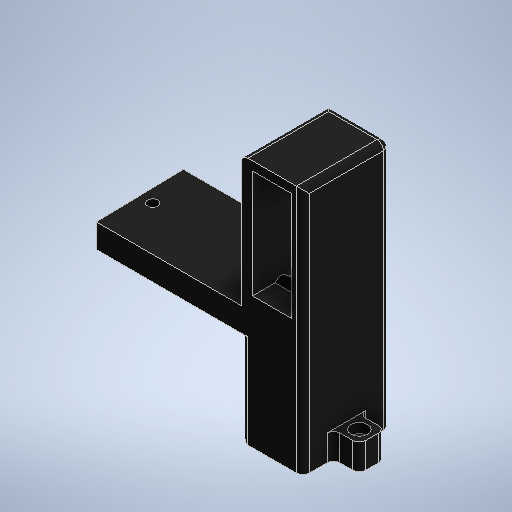
# Autodesk Inventor part: Servo Housing
Saved by Autodesk Inventor 2025.4 (Build 294407000, 407)
## iProperties
Created: 2026-05-20
Part Number: Servo Housing
Material: Generic
Document SubType Name: Modeling
Designer: lenovo
Density: 1 g/cm^3
Appearance: Default(1)
Author: lenovo
Autodesk Inventor part; units mm, degrees
ref_plane "YZ Plane" through (0, 0, 0) normal (1, 0, 0) x (0, 1, 0)
ref_plane "XZ Plane" through (0, 0, 0) normal (0, 1, 0) x (-1, 0, 0)
ref_plane "XY Plane" through (0, 0, 0) normal (0, 0, 1) x (1, 0, 0)
sketch "Sketch1" plane through (0, 0, 0) normal (0, 0, 1) x (1, 0, 0)
  line L0 (-9.5, 19.5) -> (9.5, 19.5)
  line L1 (9.5, 19.5) -> (9.5, -19.5)
  line L2 (9.5, -19.5) -> (-9.5, -19.5)
  line L3 (-9.5, -19.5) -> (-9.5, 19.5)
  line L4 (-9.5, 19.5) -> (9.5, -19.5) construction
  line L5 (9.5, 19.5) -> (-9.5, -19.5) construction
  point P0 (0, 0)
  dimension "d0" = 19
  dimension "d1" = 39
  constraints: 12 end point, 2 midpoint, 2 parallel, 1 horizontal, 1 perpendicular
  measures "d0" distance of L1.end L2.end
  measures "d1" distance of L0.end L1.end
extrude "Extrusion1" add sketch "Sketch1" along normal mid plane 27
sketch "Sketch2" plane through (0, 0, 13.5) normal (0, 0, 1) x (1, 0, 0)
  line L0 (-6.075, 16.75) -> (6.075, 16.75)
  line L1 (6.075, 16.75) -> (6.075, -16.75)
  line L2 (6.075, -16.75) -> (-6.075, -16.75)
  line L3 (-6.075, -16.75) -> (-6.075, 16.75)
  line L4 (-6.075, 16.75) -> (6.075, -16.75) construction
  line L5 (6.075, 16.75) -> (-6.075, -16.75) construction
  point P0 (0, 0)
  dimension "d4" = 12.15
  dimension "d5" = 33.5
  constraints: 12 end point, 2 midpoint, 2 parallel, 1 horizontal, 1 perpendicular
  measures "d4" distance of L1.end L2.end
  measures "d5" distance of L0.end L1.end
extrude "Extrusion2" cut sketch "Sketch2" against normal blind 7
sketch "Sketch3" plane through (0, 0, 6.5) normal (0, 0, 1) x (1, 0, 0)
  line L0 (-6.075, -16.75) -> (-6.075, 16.75) projected
  line L1 (-6.075, 0) -> (6.075, 0)
  line L2 (6.075, 16.75) -> (6.075, -16.75) projected
  circle A0 centre (0, 13.875) radius 0.625
  circle A1 centre (0, -13.875) radius 0.625
  line L3 (6.075, -16.75) -> (-6.075, -16.75) projected
  line L4 (-6.075, -16.75) -> (-4, -12.75)
  line L5 (-4, -12.75) -> (0, -12.75)
  line L6 (-6.075, 16.75) -> (6.075, 16.75) projected
  line L7 (0, 16.75) -> (0, -16.75)
  line L8 (6.075, -16.75) -> (4, -12.75)
  line L9 (4, -12.75) -> (0, -12.75)
  line L10 (-6.075, 16.75) -> (-4, 12.75)
  line L11 (-4, 12.75) -> (0, 12.75)
  line L12 (4, 12.75) -> (0, 12.75)
  line L13 (6.075, 16.75) -> (4, 12.75)
  point P0 (0, 0)
  point P1 (0, 0)
  dimension "d8" = 1.25
  dimension "d9" = 27.75
  dimension "d10" = 4
  dimension "d11" = 4
  constraints: 20 end point, 5 midpoint, 5 symmetric about line, 2 centre point, 2 vertical alignment, 1 parallel, 1 other
  measures "d8" diameter of A0
  measures "d9" diameter of A0.centre L1
  measures "d10" distance of L4.end L5.end
  measures "d11" vertical distance of L0.start L4.end
extrude "Extrusion3" cut sketch "Sketch3" against normal blind 17 contours L0 L1 L7 L5 L4 | L0 L10 L11 L7 L1 | L7 L12 L13 L2 L1 | L1 L2 L8 L9 L7 | L7 A1 | A1 L7 | L7 A0 | A0 L7
sketch "Sketch4" plane through (0, 0, -10.5) normal (0, 0, 1) x (1, 0, 0)
  line L0 (6.075, 16.75) -> (6.075, -16.75) projected
  line L1 (-6.075, -16.75) -> (6.075, -16.75)
  line L2 (6.075, -16.75) -> (6.075, 16.75)
  line L3 (6.075, 16.75) -> (-6.075, 16.75)
  line L4 (-6.075, 16.75) -> (-6.075, -16.75)
  line L5 (-6.075, -16.75) -> (6.075, 16.75) construction
  line L6 (6.075, -16.75) -> (-6.075, 16.75) construction
  point P0 (0, 0)
  constraints: 12 end point, 2 midpoint, 2 parallel, 1 horizontal, 1 perpendicular
extrude "Extrusion4" cut sketch "Sketch4" along normal blind 13
fillet "Fillet1" radius 4 4 edges at (-4, 12.75, 4.5) (4, 12.75, 4.5) (4, -12.75, 4.5) (-4, -12.75, 4.5)
sketch "Sketch5" plane through (0, 0, 13.5) normal (0, 0, 1) x (1, 0, 0)
  line L0 (9.5, -19.5) -> (-9.5, -19.5) projected
  line L1 (-9.5, -19.5) -> (9.5, -19.5)
  line L2 (9.5, -19.5) -> (9.5, -39.5)
  line L3 (9.5, -39.5) -> (-9.5, -39.5)
  line L4 (-9.5, -39.5) -> (-9.5, -19.5)
  point P0 (0, 0)
  point P1 (9.5, -29.5)
  dimension "d18" = 20
  constraints: 8 end point, 2 parallel, 1 horizontal, 1 midpoint, 1 perpendicular, 1 vertical alignment
  measures "d18" distance of L1.end L2.end
extrude "Extrusion5" add sketch "Sketch5" against normal up to surface (27 mm away)
sketch "Sketch6" plane through (-9.5, 19.5, -13.5) normal (-1, 0, 0) x (0, 0, 1)
  line L0 (27, 0) -> (27, -59) projected
  line L1 (0, 0) -> (0, -59) projected
  line L2 (27, -59) -> (27, 0) projected
  line L3 (0, -40) -> (27, -40)
  line L4 (27, -40) -> (27, -48)
  line L5 (27, -48) -> (0, -48)
  line L6 (0, -48) -> (0, -40)
  line L7 (0, 0) -> (27, 0) projected
  point P0 (13.5, -19.5)
  point P1 (27, -29.5)
  point P2 (0, -48)
  dimension "d28" = 8
  dimension "d29" = 40
  constraints: 8 end point, 2 parallel, 2 point on line, 1 horizontal, 1 midpoint, 1 perpendicular
  measures "d28" distance between parallel lines of L3 L5
  measures "d29" distance between parallel lines of L7 L3
extrude "Extrusion6" add sketch "Sketch6" along normal blind 45 contours L0 L5 L1 L3
sketch "Sketch7" plane through (9.5, -39.5, -13.5) normal (0, -1, 0) x (1, 0, 0)
  line L0 (0, 0) -> (0, 27) projected
  line L1 (0, 27) -> (-19, 27)
  line L2 (-19, 27) -> (-19, 0)
  line L3 (-19, 0) -> (0, 0)
  line L4 (0, 0) -> (0, 27)
  point P0 (-9.5, 13.5)
  constraints: 8 end point, 2 parallel, 1 horizontal, 1 perpendicular
extrude "Extrusion7" add sketch "Sketch7" along normal blind 18
sketch "Sketch8" plane through (9.5, -57.5, -13.5) normal (0, -1, 0) x (1, 0, 0)
  line L0 (-15.575, 16) -> (-15.575, 3) projected
  line L1 (-3.425, 16) -> (-15.575, 16) projected
  line L2 (-15.575, 3) -> (-3.425, 3)
  line L3 (-3.425, 3) -> (-3.425, 16)
  line L4 (-3.425, 16) -> (-15.575, 16)
  line L5 (-15.575, 16) -> (-15.575, 3)
  point P0 (-9.5, 13.5)
  constraints: 8 end point, 2 parallel, 1 horizontal, 1 perpendicular
extrude "Extrusion8" cut sketch "Sketch8" against normal up to next
sketch "Sketch9" plane through (9.5, -57.5, -13.5) normal (0, -1, 0) x (1, 0, 0)
  line L0 (0, 0) -> (0, 27) projected
  line L1 (0, 17.5) -> (8, 17.5)
  line L2 (8, 17.5) -> (8, 9.5)
  line L3 (8, 9.5) -> (0, 9.5)
  line L4 (0, 9.5) -> (0, 17.5)
  circle A0 centre (4, 13.5) radius 1.6
  line L5 (-15.575, 16) -> (-3.425, 16) projected
  line L6 (-9.5, 16) -> (-9.5, 3)
  line L7 (-3.425, 3) -> (-15.575, 3) projected
  line L8 (-19, 17.5) -> (-27, 17.5)
  line L9 (-27, 17.5) -> (-27, 9.5)
  line L10 (-27, 9.5) -> (-19, 9.5)
  circle A1 centre (-23, 13.5) radius 1.6
  line L11 (-19, 17.5) -> (-19, 9.5)
  point P0 (-9.5, 13.5)
  point P1 (8, 13.5)
  point P2 (0, 13.5)
  point P3 (4, 17.5)
  point P4 (0, 9.5)
  dimension "d30" = 8
  dimension "d31" = 8
  dimension "d32" = 3.2
  constraints: 18 end point, 5 midpoint, 5 symmetric about line, 2 centre point, 2 horizontal alignment, 2 parallel, 2 perpendicular, 1 horizontal, 1 point on line, 1 vertical alignment, 1 other
  measures "d30" distance of L1.start L1.end
  measures "d31" distance between parallel lines of L1 L3
  measures "d32" diameter of A0
extrude "Extrusion9" add sketch "Sketch9" against normal blind 8
sketch "Sketch10" plane through (9.5, -49.5, -13.5) normal (0, 1, 0) x (1, 0, 0)
  circle A0 centre (4, -13.5) radius 1.6 projected
  circle A1 centre (4, -13.5) radius 2.6
  circle A2 centre (-23, -13.5) radius 2.6
  circle A3 centre (-23, -13.5) radius 1.6 projected
  point P0 (-9.5, -13.5)
  dimension "d35" = 5.2
  dimension "d36" = 5.2
  constraints: 2 centre point, 1 coincident, 1 concentric
  measures "d35" diameter of A1
  measures "d36" diameter of A2
extrude "Extrusion10" cut sketch "Sketch10" against normal blind 3
fillet "Fillet2" radius 2 15 edges at (-9.5, -43, 13.5) (9.5, -19, 13.5) (9.5, -53.5, 4) (17.5, -53.5, 4) (17.5, -53.5, -4) (9.5, -53.5, -4) (6.075, -20.375, -10.5) (-9.5, -43, -13.5) (-9.5, -53.5, -4) (-17.5, -53.5, -4) (-17.5, -53.5, 4) (-9.5, -53.5, 4) (9.5, 19.5, 0) (-9.5, 19.5, 0) (0, 19.5, -13.5)
fillet "Fillet3" radius 2 2 edges at (8.9142, 18.9142, -12.9142) (9.5, -20, -13.5)
sketch "Sketch12" plane through (-54.5, 19.5, -13.5) normal (-1, 0, 0) x (0, 0, 1)
  line L0 (0, -40) -> (0, -48) projected
  line L1 (0, -40) -> (27, -40.5939)
  line L2 (27, -48) -> (27, -40) projected
  line L3 (27, -40) -> (0, -40) projected
  point P0 (13.5, -19.5)
  dimension "d47" = 1.26
  constraints: 2 end point, 1 point on line
  measures "d47" angle of L3 L1
extrude "Extrusion12" cut sketch "Sketch12" against normal up to surface (45 mm away)
sketch "Sketch13" plane through (-54.5, -20.5, -13.5) normal (0, 0.9997582, 0.0219894) x (1, 0, 0)
  circle A0 centre (4, -13.5033) radius 1.6
  line L0 (0, -27.0065) -> (0, 0) projected
  circle A1 centre (34, -13.5033) radius 1.6
  point P0 (54.5, -13.046)
  point P1 (0, -13.5033)
  dimension "d50" = 3.2
  dimension "d51" = 4
  dimension "d52" = 3.2
  dimension "d53" = 30
  constraints: 2 centre point, 2 horizontal alignment, 1 midpoint
  measures "d50" diameter of A0
  measures "d51" distance from line of L0 A0.centre
  measures "d52" diameter of A1
  measures "d53" distance of A0.centre A1.centre
extrude "Extrusion13" cut sketch "Sketch13" against normal up to next
equation "\"d31\" = d30"
body "Solid1"
